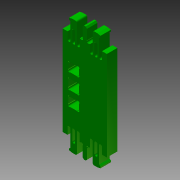
# Autodesk Inventor part: floor_back
Saved by Autodesk Inventor 2012 SP1 (Build 160190100, 190)
## iProperties
Created: 2011-10-14
Part Number: floor_back
Document SubType Name: Modeling
Designer: cramera
Density: 0.952 g/cm^3
Material: High Density Polyethylene
Mass: 57.2271 g
Surface Area: 209.442 cm^2
Volume: 60.1125 cm^3
Autodesk Inventor part; units mm, degrees
ref_plane "YZ Plane" through (0, 0, 0) normal (1, 0, 0) x (0, 1, 0)
ref_plane "XZ Plane" through (0, 0, 0) normal (0, 1, 0) x (-1, 0, 0)
ref_plane "XY Plane" through (0, 0, 0) normal (0, 0, 1) x (1, 0, 0)
derived "skeleton.ipt"
sketch "STOCK_12MM" plane through (0, 0, 0) normal (0, 0, 1) x (1, 0, 0)
  line L0 (457.2, 914.4) -> (457.2, 0)
  line L1 (0, 0) -> (457.2, 0)
  line L2 (457.2, 0) -> (457.2, 914.4)
  line L3 (457.2, 914.4) -> (0, 914.4)
  line L4 (0, 914.4) -> (0, 0)
  constraints: 10 end point
sketch "THROUGH-CUT" plane through (0, 0, 0) normal (0, 0, 1) x (1, 0, 0)
  arc A0 (342.5261, 144.4847) -> (340.281, 142.2396) centre (341.4036, 143.3622) ccw
  line L0 (340.281, 142.2396) -> (340.281, 136.5697)
  arc A1 (340.281, 136.5697) -> (342.5261, 134.3247) centre (341.4036, 135.4472) ccw
  line L1 (342.5261, 134.3247) -> (350.355, 134.3247)
  arc A2 (350.355, 134.3247) -> (352.6, 136.5697) centre (351.4775, 135.4472) ccw
  line L2 (352.6, 136.5697) -> (352.6, 142.2396)
  arc A3 (352.6, 142.2396) -> (350.355, 144.4847) centre (351.4775, 143.3622) ccw
  line L3 (350.355, 144.4847) -> (342.5261, 144.4847)
  line L4 (350.355, 99.7807) -> (342.5261, 99.7807)
  arc A4 (340.281, 102.0257) -> (342.5261, 99.7807) centre (341.4036, 100.9032) ccw
  line L5 (340.281, 102.0257) -> (340.281, 107.6956)
  arc A5 (342.5261, 109.9407) -> (340.281, 107.6956) centre (341.4036, 108.8182) ccw
  line L6 (342.5261, 109.9407) -> (350.355, 109.9407)
  arc A6 (352.6, 107.6956) -> (350.355, 109.9407) centre (351.4775, 108.8182) ccw
  line L7 (352.6, 107.6956) -> (352.6, 102.0257)
  arc A7 (350.355, 99.7807) -> (352.6, 102.0257) centre (351.4775, 100.9032) ccw
  line L8 (350.355, 116.4177) -> (342.5261, 116.4177)
  arc A8 (340.281, 118.6627) -> (342.5261, 116.4177) centre (341.4036, 117.5402) ccw
  line L9 (340.281, 118.6627) -> (340.281, 125.6026)
  arc A9 (342.5261, 127.8477) -> (340.281, 125.6026) centre (341.4036, 126.7252) ccw
  line L10 (342.5261, 127.8477) -> (350.355, 127.8477)
  arc A10 (352.6, 125.6026) -> (350.355, 127.8477) centre (351.4775, 126.7252) ccw
  line L11 (352.6, 125.6026) -> (352.6, 118.6627)
  arc A11 (350.355, 116.4177) -> (352.6, 118.6627) centre (351.4775, 117.5402) ccw
  arc A12 (372.0945, 178.9049) -> (370.507, 177.3174) centre (372.0945, 177.3174) ccw
  line L12 (372.0945, 178.9049) -> (372.2215, 178.9049)
  arc A13 (373.809, 177.3174) -> (372.2215, 178.9049) centre (372.2215, 177.3174) ccw
  line L13 (373.809, 177.3174) -> (373.809, 165.7889)
  arc A14 (372.2215, 164.2014) -> (373.809, 165.7889) centre (372.2215, 165.7889) ccw
  line L14 (372.2215, 164.2014) -> (372.0945, 164.2014)
  arc A15 (370.507, 165.7889) -> (372.0945, 164.2014) centre (372.0945, 165.7889) ccw
  line L15 (370.507, 165.7889) -> (370.507, 177.3174)
  arc A16 (344.853, 66.948) -> (346.4405, 65.3605) centre (346.4405, 66.948) ccw
  line L16 (344.853, 66.948) -> (344.853, 78.4764)
  arc A17 (346.4405, 80.0639) -> (344.853, 78.4764) centre (346.4405, 78.4764) ccw
  line L17 (346.4405, 80.0639) -> (346.5675, 80.0639)
  arc A18 (348.155, 78.4764) -> (346.5675, 80.0639) centre (346.5675, 78.4764) ccw
  line L18 (348.155, 78.4764) -> (348.155, 66.948)
  arc A19 (346.5675, 65.3605) -> (348.155, 66.948) centre (346.5675, 66.948) ccw
  line L19 (346.5675, 65.3605) -> (346.4405, 65.3605)
  arc A20 (348.155, 177.3174) -> (346.5675, 178.9049) centre (346.5675, 177.3174) ccw
  line L20 (346.5675, 178.9049) -> (346.4405, 178.9049)
  arc A21 (346.4405, 178.9049) -> (344.853, 177.3174) centre (346.4405, 177.3174) ccw
  line L21 (344.853, 177.3174) -> (344.853, 165.7889)
  arc A22 (344.853, 165.7889) -> (346.4405, 164.2014) centre (346.4405, 165.7889) ccw
  line L22 (346.4405, 164.2014) -> (346.5675, 164.2014)
  arc A23 (346.5675, 164.2014) -> (348.155, 165.7889) centre (346.5675, 165.7889) ccw
  line L23 (348.155, 165.7889) -> (348.155, 177.3174)
  line L24 (375.841, 165.7889) -> (375.841, 182.5292)
  line L25 (375.841, 182.5292) -> (375.841, 185.1564)
  line L26 (375.841, 185.1564) -> (377.365, 186.4264)
  line L27 (377.365, 186.4264) -> (377.365, 188.1444)
  line L28 (377.365, 188.1444) -> (373.7655, 188.9664)
  line L29 (373.7655, 188.9664) -> (370.0604, 188.9664)
  arc A24 (370.0604, 188.9664) -> (368.475, 187.3789) centre (370.0625, 187.3789) ccw
  line L30 (368.475, 187.3789) -> (368.475, 165.7889)
  arc A25 (366.8875, 164.2014) -> (368.475, 165.7889) centre (366.8875, 165.7889) ccw
  line L31 (366.8875, 164.2014) -> (366.7605, 164.2014)
  arc A26 (365.173, 165.7889) -> (366.7605, 164.2014) centre (366.7605, 165.7889) ccw
  line L32 (365.173, 165.7889) -> (365.173, 173.7264)
  line L33 (365.173, 173.7264) -> (364.1161, 173.7264)
  arc A27 (361.871, 175.9715) -> (364.1161, 173.7264) centre (362.9936, 174.849) ccw
  line L34 (361.871, 175.9715) -> (361.871, 187.3789)
  line L35 (361.871, 187.3789) -> (360.2835, 188.9664)
  line L36 (360.2835, 188.9664) -> (358.3785, 188.9664)
  line L37 (358.3785, 188.9664) -> (356.791, 187.3789)
  line L38 (356.791, 187.3789) -> (356.791, 175.9715)
  arc A28 (356.791, 173.7264) -> (356.791, 175.9715) centre (355.6685, 174.849) ccw
  arc A29 (354.546, 173.7264) -> (356.791, 173.7264) centre (355.6685, 174.849) ccw
  line L39 (354.546, 173.7264) -> (353.489, 173.7264)
  line L40 (353.489, 173.7264) -> (353.489, 165.7889)
  arc A30 (351.9015, 164.2014) -> (353.489, 165.7889) centre (351.9015, 165.7889) ccw
  line L41 (351.9015, 164.2014) -> (351.7745, 164.2014)
  arc A31 (350.187, 165.7889) -> (351.7745, 164.2014) centre (351.7745, 165.7889) ccw
  line L42 (350.187, 165.7889) -> (350.187, 187.3789)
  arc A32 (350.187, 187.3789) -> (348.5995, 188.9664) centre (348.5995, 187.3789) ccw
  line L43 (348.5995, 188.9664) -> (344.8966, 188.9664)
  line L44 (344.8966, 188.9664) -> (341.297, 188.1444)
  line L45 (341.297, 188.1444) -> (341.297, 186.4264)
  line L46 (341.297, 186.4264) -> (342.821, 185.1564)
  line L47 (342.821, 185.1564) -> (342.821, 182.5292)
  line L48 (342.821, 182.5292) -> (342.821, 165.7889)
  arc A33 (341.2335, 164.2014) -> (342.821, 165.7889) centre (341.2335, 165.7889) ccw
  line L49 (341.2335, 164.2014) -> (341.1065, 164.2014)
  arc A34 (339.519, 165.7889) -> (341.1065, 164.2014) centre (341.1065, 165.7889) ccw
  line L50 (339.519, 165.7889) -> (339.519, 173.7264)
  line L51 (339.519, 173.7264) -> (333.931, 173.7264)
  line L52 (333.931, 173.7264) -> (333.931, 70.5389)
  line L53 (333.931, 70.5389) -> (339.519, 70.5389)
  line L54 (339.519, 70.5389) -> (339.519, 78.4764)
  arc A35 (341.1065, 80.0639) -> (339.519, 78.4764) centre (341.1065, 78.4764) ccw
  line L55 (341.1065, 80.0639) -> (341.2335, 80.0639)
  arc A36 (342.821, 78.4764) -> (341.2335, 80.0639) centre (341.2335, 78.4764) ccw
  line L56 (342.821, 78.4764) -> (342.821, 61.7362)
  line L57 (342.821, 61.7362) -> (342.821, 59.1089)
  line L58 (342.821, 59.1089) -> (341.297, 57.8389)
  line L59 (341.297, 57.8389) -> (341.297, 56.121)
  line L60 (341.297, 56.121) -> (344.8966, 55.2989)
  line L61 (344.8966, 55.2989) -> (348.5995, 55.2989)
  arc A37 (348.5995, 55.2989) -> (350.187, 56.8864) centre (348.5995, 56.8864) ccw
  line L62 (350.187, 56.8864) -> (350.187, 78.4764)
  arc A38 (351.7745, 80.0639) -> (350.187, 78.4764) centre (351.7745, 78.4764) ccw
  line L63 (351.7745, 80.0639) -> (351.9015, 80.0639)
  arc A39 (353.489, 78.4764) -> (351.9015, 80.0639) centre (351.9015, 78.4764) ccw
  line L64 (353.489, 78.4764) -> (353.489, 70.5389)
  line L65 (353.489, 70.5389) -> (354.546, 70.5389)
  arc A40 (356.791, 68.2939) -> (354.546, 70.5389) centre (355.6685, 69.4164) ccw
  line L66 (356.791, 68.2939) -> (356.791, 56.8864)
  line L67 (356.791, 56.8864) -> (358.3785, 55.2989)
  line L68 (358.3785, 55.2989) -> (360.2835, 55.2989)
  line L69 (360.2835, 55.2989) -> (361.871, 56.8864)
  line L70 (361.871, 56.8864) -> (361.871, 68.2939)
  arc A41 (364.1161, 70.5389) -> (361.871, 68.2939) centre (362.9936, 69.4164) ccw
  line L71 (364.1161, 70.5389) -> (365.173, 70.5389)
  line L72 (365.173, 70.5389) -> (365.173, 78.4764)
  arc A42 (366.7711, 80.0639) -> (365.173, 78.4764) centre (366.7605, 78.4764) ccw
  line L73 (366.7711, 80.0639) -> (366.8875, 80.0639)
  arc A43 (368.475, 78.4764) -> (366.8875, 80.0639) centre (366.8875, 78.4764) ccw
  line L74 (368.475, 78.4764) -> (368.475, 56.8864)
  arc A44 (368.475, 56.8864) -> (370.0604, 55.2989) centre (370.0625, 56.8864) ccw
  line L75 (370.0604, 55.2989) -> (373.7655, 55.2989)
  line L76 (373.7655, 55.2989) -> (377.365, 56.121)
  line L77 (377.365, 56.121) -> (377.365, 57.8389)
  line L78 (377.365, 57.8389) -> (375.841, 59.1089)
  line L79 (375.841, 59.1089) -> (375.841, 61.7362)
  line L80 (375.841, 61.7362) -> (375.841, 78.4764)
  arc A45 (377.4285, 80.0639) -> (375.841, 78.4764) centre (377.4285, 78.4764) ccw
  line L81 (377.4285, 80.0639) -> (377.5555, 80.0639)
  arc A46 (379.143, 78.4764) -> (377.5555, 80.0639) centre (377.5555, 78.4764) ccw
  line L82 (379.143, 78.4764) -> (379.143, 70.5389)
  line L83 (379.143, 70.5389) -> (384.731, 70.5389)
  line L84 (384.731, 70.5389) -> (384.731, 173.7264)
  line L85 (384.731, 173.7264) -> (379.143, 173.7264)
  line L86 (379.143, 173.7264) -> (379.143, 165.7889)
  arc A47 (377.5555, 164.2014) -> (379.143, 165.7889) centre (377.5555, 165.7889) ccw
  line L87 (377.5555, 164.2014) -> (377.4285, 164.2014)
  arc A48 (375.841, 165.7889) -> (377.4285, 164.2014) centre (377.4285, 165.7889) ccw
  arc A49 (370.507, 66.948) -> (372.0945, 65.3605) centre (372.0945, 66.948) ccw
  line L88 (372.0945, 65.3605) -> (372.2215, 65.3605)
  arc A50 (372.2215, 65.3605) -> (373.809, 66.948) centre (372.2215, 66.948) ccw
  line L89 (373.809, 66.948) -> (373.809, 78.4764)
  arc A51 (373.809, 78.4764) -> (372.2215, 80.0639) centre (372.2215, 78.4764) ccw
  line L90 (372.2215, 80.0639) -> (372.0945, 80.0639)
  arc A52 (372.0945, 80.0639) -> (370.507, 78.4764) centre (372.0945, 78.4764) ccw
  line L91 (370.507, 78.4764) -> (370.507, 66.948)
  constraints: 184 end point, 106 point on circle, 53 centre point
extrude "Extrusion1" add sketch "THROUGH-CUT" along normal blind 12
equation "\"d1\" = StockThickness"
equation "\"StockThickness\" = 12"
body "Solid1"
